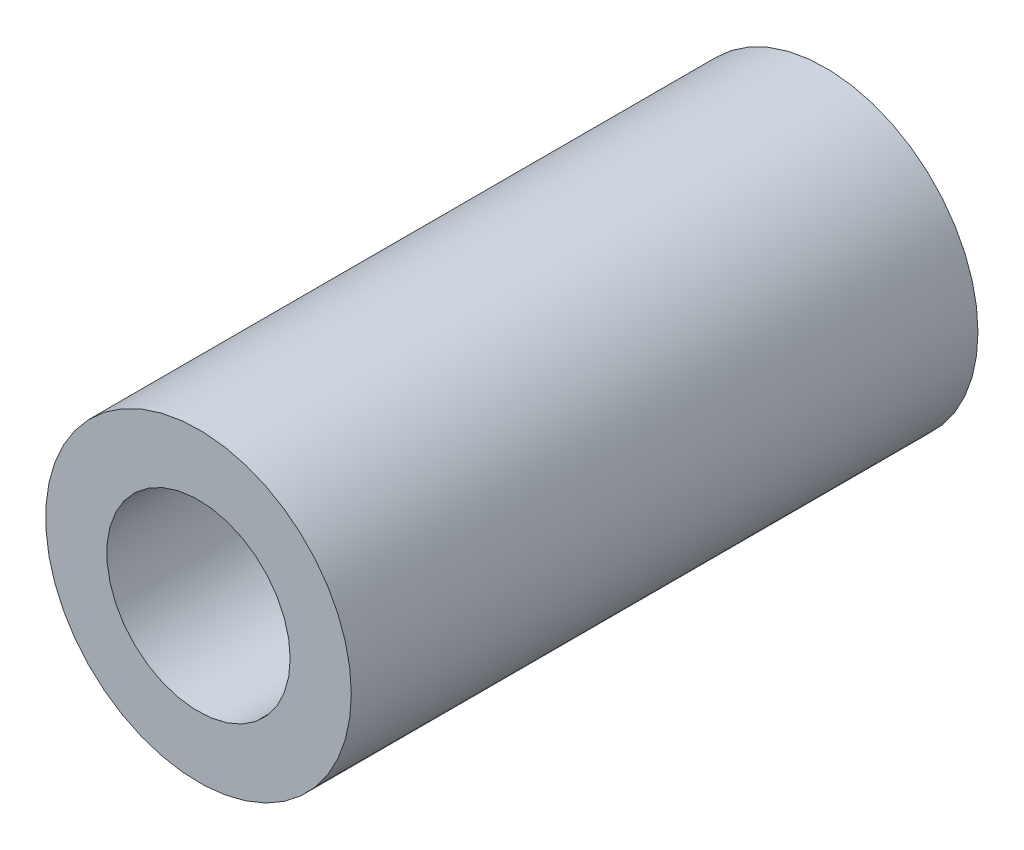
# Autodesk Inventor part: Upper Connecting Standoff
Saved by Autodesk Inventor 2014 SP1 (Build 180222100, 222)
## iProperties
Created: 2014-01-10
Part Number: Upper Connecting Standoff
Material: Aluminum 6061
Document SubType Name: Modeling
Designer: Rauhul Varma
Mass: 11.1721 g
Surface Area: 28.5023 cm^2
Volume: 4.12254 cm^3
Density: 2.71 g/cm^3
Appearance: Anodized - Black
Author: Rauhul Varma
Autodesk Inventor part; units mm, degrees
ref_plane "YZ Plane" through (0, 0, 0) normal (1, 0, 0) x (0, 1, 0)
ref_plane "XZ Plane" through (0, 0, 0) normal (0, 1, 0) x (-1, 0, 0)
ref_plane "XY Plane" through (0, 0, 0) normal (0, 0, 1) x (1, 0, 0)
sketch "Sketch1" plane through (0, 0, 0) normal (0, 0, 1) x (1, 0, 0)
  circle A0 centre (0, 0) radius 7.9375
  circle A1 centre (0, 0) radius 4.7625
  dimension "d0" = 15.875
  dimension "d1" = 9.525
  constraints: 2 centre point, 2 coincident
  measures "d0" diameter of A0
  measures "d1" diameter of A1
extrude "Extrusion1" add sketch "Sketch1" along normal blind 32.5438
body "Solid1"
